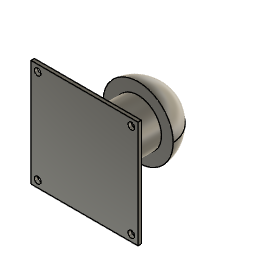
Suport+Topo+V2 (Autodesk Fusion 360 archive; units mm, degrees)
design "camera"
Autodesk Fusion 360 part; units mm, degrees
sketch "Sketch1" plane through (0, 0, 0) normal (0, 1, 0) x (1, 0, 0)
  line L0 (0, 0) -> (32, 0)
  line L1 (32, 0) -> (32, -32)
  line L2 (32, -32) -> (0, -32)
  line L3 (0, -32) -> (0, 0)
  circle A0 centre (1.6953, -30.2758) radius 1.5
  circle A1 centre (1.6953, -1.6758) radius 1.5
  circle A2 centre (30.3047, -30.2758) radius 1.5
  circle A3 centre (30.3047, -1.6758) radius 1.5
  line L4 (-1, -16) -> (38, -16)
  line L5 (0, -13) -> (9.5, -13)
  line L6 (32, -13) -> (22.5, -13)
  line L7 (9.5, 0.8661) -> (9.5, -33)
  line L8 (22.5, 0.9345) -> (22.5, -33)
  line L9 (16, 2.2342) -> (16, -35)
  line L10 (22.5, -9.5) -> (9.5, -9.5)
  line L11 (9.5, -9.5) -> (9.5, -22.5)
  line L12 (9.5, -22.5) -> (22.5, -22.5)
  line L13 (22.5, -22.5) -> (22.5, -9.5)
  line L14 (22.5, -9.5) -> (9.5, -22.5) construction
  line L15 (9.5, -9.5) -> (22.5, -22.5) construction
  circle A4 centre (16, -16) radius 6.5
  line L16 (0, 1) -> (10, 1)
  line L17 (32, 1) -> (20, 1)
  line L18 (10, 1) -> (10, -6)
  line L19 (20, 1) -> (20, -6)
  line L20 (10, -5.4961) -> (20, -5.4961)
  line L21 (20, -5.4961) -> (20, -0.4961)
  line L22 (20, -0.4961) -> (10, -0.4961)
  line L23 (10, -0.4961) -> (10, -5.4961)
  line L24 (24.5, -14) -> (22.5, -14)
  line L25 (22.5, -14) -> (22.5, -18)
  line L26 (22.5, -18) -> (24.5, -18)
  line L27 (24.5, -18) -> (24.5, -14)
  arc A5 (24.5, -18) -> (24.5, -14) centre (24.5, -16) ccw
  arc A6 (22.5, -15.9983) -> (22.5, -16.0017) centre (24.5, -16) ccw
  arc A7 (7.5, -14) -> (7.5, -18) centre (7.5, -16) ccw
  line L28 (7.5, -14) -> (9.5, -14)
  line L29 (9.5, -18) -> (7.5, -18)
  point P0 (16, -16)
  constraint horizontal L0
  constraint vertical L1
  constraint horizontal L2
  constraint vertical L3
  constraint coincident L0.start L3.end
  constraint coincident L3 L5.start
  constraint perpendicular L3 L5
  constraint coincident L1 L6.start
  constraint perpendicular L1 L6
  constraint perpendicular L2 L7
  constraint perpendicular L2 L8
  constraint perpendicular L2 L9
  constraint horizontal L10
  constraint perpendicular L10 L11
  constraint parallel L10 L12
  constraint parallel L11 L13
  constraint coincident L14 P0
  constraint coincident L15 P0
  constraint coincident L4 P0
  constraint coincident L9 P0
  constraint coincident P0 A4.centre
  constraint tangent L13 A4
  constraint perpendicular L3 L16
  constraint perpendicular L8 L17
  constraint perpendicular L0 L18
  constraint perpendicular L0 L19
  constraint horizontal L20
  constraint vertical L21
  constraint horizontal L22
  constraint vertical L23
  constraint coincident L18 L20.start
  constraint horizontal L24
  constraint vertical L25
  constraint horizontal L26
  constraint vertical L27
  constraint midpoint L27 A5.centre
  constraint coincident L8 A6.end
  constraint coincident L8 A6.start
  constraint concentric A5 A6
  constraint symmetric L9 L24.start A7.start
  constraint symmetric L9 L24.end L28.end
  constraint symmetric L9 L25.end L29.start
  constraint symmetric L9 L26.end A7.end
  constraint symmetric L9 A5 A7
extrude "Extrude1" add sketch "Sketch1" against normal blind 3 makes body 1
extrude "Extrude2" add sketch "Sketch1" along normal blind 12.5 contours L9 L18 L20 L22 L23 | L9 L19 L20 L21 L22 bodies 1
extrude "Extrude3" add sketch "Sketch1" against normal blind 6 contours L7 L10 L11 A4 | L4 L9 A4 | L8 L10 L13 A4 L25 | L4 L9 A4 | L4 L7 L11 A7 L28 | L4 L7 L11 A7 L29 | L4 L9 A4 | L4 L9 A4 | L4 L8 L13 L24 L25 L27 | L4 L8 L13 L25 L26 L27 | L8 L12 L13 A4 L25 | L7 L11 L12 A4 | L4 L27 A5 | L4 L27 A5 bodies 1
extrude "Extrude4" add sketch "Sketch1" against normal blind 18.4 contours L4 L9 A4 | L4 L9 A4 | L4 L9 A4 | L4 L9 A4 bodies 1
sketch "Sketch2" plane through (0, 0, 0) normal (0, 1, 0) x (1, 0, 0)
  circle A0 through (26.5, -16, -18.3) (10.75, -6.9067, -18.3) (10.75, -25.0933, -18.3)
extrude "Extrude5" add sketch "Sketch2" against normal blind 11 contours A0 in plane through (0, -18.3, 0) normal (0, 1, 0) bodies 1
sketch "Sketch3" plane through (0, 0, 0) normal (0, 1, 0) x (1, 0, 0)
  line L0 (0, 0) -> (-16, 0)
  line L1 (-16, 0) -> (-16, -16)
  line L2 (0, 0) -> (-32, 0)
  line L3 (-32, 0) -> (-32, -32)
  line L4 (-32, -32) -> (0, -32)
  line L5 (0, -32) -> (0, 0)
  line L6 (0, 0) -> (-32, -32) construction
  line L7 (-32, 0) -> (0, -32) construction
  line L8 (0, 0) -> (-2, 0)
  line L9 (-2, 0) -> (-2, -2)
  circle A0 centre (-2, -2) radius 1
  circle A1 centre (-30, -2) radius 1
  circle A2 centre (-30, -30) radius 1
  circle A3 centre (-2, -30) radius 1
  circle A4 centre (-16, -16) radius 7
  line L10 (-22.5, -9.5) -> (-9.5, -9.5)
  line L11 (-9.5, -9.5) -> (-9.5, -22.5)
  line L12 (-9.5, -22.5) -> (-22.5, -22.5)
  line L13 (-22.5, -22.5) -> (-22.5, -9.5)
  line L14 (-22.5, -9.5) -> (-9.5, -22.5) construction
  line L15 (-9.5, -9.5) -> (-22.5, -22.5) construction
  line L16 (-25.5, -14) -> (-18.5, -14)
  line L17 (-18.5, -14) -> (-18.5, -18)
  line L18 (-18.5, -18) -> (-25.5, -18)
  line L19 (-26.5, -17) -> (-26.5, -15)
  line L20 (-26.5, -14) -> (-18.5, -18) construction
  line L21 (-18.5, -14) -> (-26.5, -18) construction
  arc A5 (-26.5, -17) -> (-25.5, -18) centre (-25.5, -17) ccw
  arc A6 (-25.5, -14) -> (-26.5, -15) centre (-25.5, -15) ccw
  line L22 (-6.5, -18) -> (-13.5, -18)
  line L23 (-13.5, -18) -> (-13.5, -14)
  line L24 (-13.5, -14) -> (-6.5, -14)
  line L25 (-5.5, -15) -> (-5.5, -17)
  line L26 (-5.5, -18) -> (-13.5, -14) construction
  line L27 (-13.5, -18) -> (-5.5, -14) construction
  arc A7 (-6.5, -18) -> (-5.5, -17) centre (-6.5, -17) ccw
  arc A8 (-5.5, -15) -> (-6.5, -14) centre (-6.5, -15) ccw
  point P0 (-16, -16)
  point P1 (-16, -16)
  point P2 (-22.5, -16)
  point P3 (-9.5, -16)
  dimension "d25" = 16
  dimension "d26" = 16
  dimension "d27" = 2
  dimension "d28" = 2
  dimension "d30" = 360
  dimension "d31" = 14
  dimension "d32" = 13
  dimension "d33" = 13
  dimension "d34" = 8
  dimension "d35" = 4
  dimension "d40" = 1
  dimension "d41" = 1
  dimension "d53" = 8
  dimension "d54" = 4
  dimension "d55" = 1
  dimension "d56" = 1
  constraint coincident L0.start L2.start
  constraint horizontal L0
  constraint perpendicular L0 L1
  constraint horizontal L2
  constraint perpendicular L2 L3
  constraint parallel L2 L4
  constraint parallel L3 L5
  constraint coincident L6 P1
  constraint coincident L7 P1
  constraint coincident P1 P0
  constraint parallel L0 L8
  constraint coincident L6 L9.end
  constraint perpendicular L2 L9
  constraint coincident L9.end A0.centre
  constraint horizontal L10
  constraint perpendicular L10 L11
  constraint parallel L10 L12
  constraint parallel L11 L13
  constraint coincident L14 P1
  constraint coincident L15 P1
  constraint horizontal L16
  constraint perpendicular L16 L17
  constraint parallel L16 L18
  constraint parallel L17 L19
  constraint coincident L20 P2
  constraint coincident L21 P2
  constraint midpoint L13 P2
  constraint coincident L21.end L18
  constraint coincident L21.end L19
  constraint tangent L18 A5
  constraint tangent L19 A5
  constraint coincident L20.start L19
  constraint coincident L20.start L16
  constraint tangent L19 A6
  constraint tangent L16 A6
  constraint horizontal L22
  constraint perpendicular L22 L23
  constraint parallel L22 L24
  constraint parallel L23 L25
  constraint coincident L26 P3
  constraint coincident L27 P3
  constraint midpoint L11 P3
  constraint coincident L26.start L22
  constraint coincident L26.start L25
  constraint tangent L22 A7
  constraint tangent L25 A7
  constraint coincident L27.end L24
  constraint coincident L27.end L25
  constraint tangent L24 A8
  constraint tangent L25 A8
  measures "d25" distance of L0.start L0.end
  measures "d26" distance of L0.end P1
  measures "d27" distance of L0.start L8.end
  measures "d28" diameter of A0
  measures "d31" diameter of A4
  measures "d32" distance of L11.end L12.end
  measures "d33" distance of L10.end L11.end
  measures "d34" distance of L17.end L21.end
  measures "d35" distance of L16.end L17.end
  measures "d40" radius of A5
  measures "d41" radius of A6
  measures "d53" distance of L23.end L27.end
  measures "d54" distance of L22.end L23.end
  measures "d55" radius of A7
  measures "d56" radius of A8
extrude "Extrude6" add sketch "Sketch3" along normal blind 1 separate body contours L0 L2 L3 L4 L5 L8 | L1 A4 L10 | L1 A4 L10 | A4 L10 L11 L12 L13 L16 L17 L18 L22 L23 L24 | A4 L10 L11 | A4 L10 L13 | A4 L11 L24 | A4 L13 L16 | A4 L22 L24 L25 A7 A8 | A4 L11 L22 L24 | L11 L22 L23 L24 | A4 L13 L16 L18 | A4 L16 L18 L19 A5 A6 | L13 L16 L17 L18 | A4 L11 L22 | A4 L13 L18 | A4 L11 L12 | A4 L12 L13 | A4 L12 makes body 2
extrude "Extrude7" add sketch "Sketch3" against normal blind 3 contours L1 A4 L10 | L1 A4 L10 | A4 L10 L11 L12 L13 L16 L17 L18 L22 L23 L24 | A4 L10 L11 | A4 L10 L13 | A4 L11 L24 | A4 L13 L16 | A4 L22 L24 L25 A7 A8 | A4 L11 L22 L24 | L11 L22 L23 L24 | A4 L13 L16 L18 | A4 L16 L18 L19 A5 A6 | L13 L16 L17 L18 | A4 L11 L22 | A4 L13 L18 | A4 L11 L12 | A4 L12 L13 | A4 L12 bodies 2
extrude "Extrude8" add sketch "Sketch3" against normal blind 15 contours L1 A4 L10 | L1 A4 L10 | A4 L10 L11 L12 L13 L16 L17 L18 L22 L23 L24 | A4 L11 L24 | A4 L13 L16 | A4 L11 L22 L24 | L11 L22 L23 L24 | A4 L13 L16 L18 | L13 L16 L17 L18 | A4 L11 L22 | A4 L13 L18 | A4 L12 bodies 2
sketch "Sketch4" plane through (0, -15, 0) normal (0, -1, 0) x (1, 0, 0)
  circle A0 centre (-16, 16) radius 7
  circle A1 centre (-16, 16) radius 10.5
  dimension "d48" = 21
  constraint concentric A0 A1
  measures "d48" diameter of A1
extrude "Extrude9" add sketch "Sketch4" along normal blind 10 contours A0 | A1 bodies 2
fillet "Fillet1" radius 10 tangency weight 0.79029 1 edges at (-25.7894, -25, 12.203) on bodies 2
move_body "Move1" bodies 2 to x (-1, 0, 0) y (0, -1, 0) z (0, 0, 1) at (0, 1, 0)
hidden bodies 1
equation "d25 = ( 32 / 2 ) * 1 mm"
equation "d26 = ( 32 / 2 ) * 1 mm"

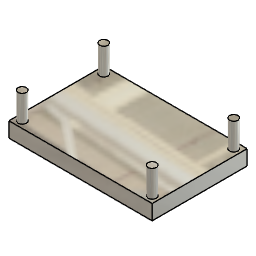
design "ecra Pi Pico"
Autodesk Fusion 360 part; units mm, degrees
sketch "Sketch1" plane through (0, 0, 0) normal (0, 1, 0) x (1, 0, 0)
  line L0 (43, -28.5) -> (-43, -28.5)
  line L1 (-43, -28.5) -> (-43, 28.5)
  line L2 (-43, 28.5) -> (43, 28.5)
  line L3 (43, 28.5) -> (43, -28.5)
  line L4 (43, -28.5) -> (-43, 28.5) construction
  line L5 (-43, -28.5) -> (43, 28.5) construction
  line L6 (43, -28.5) -> (39, -28.5)
  line L7 (39, -28.5) -> (39, -24.5)
  line L8 (39, -24.5) -> (43, -24.5)
  line L9 (43, -24.5) -> (43, -28.5)
  circle A0 centre (39, -24.5) radius 2.5
  line L10 (52.3114, 0) -> (-55.6196, 0)
  line L11 (0, 36.5366) -> (0, -32.8551)
  circle A1 centre (-39, -24.5) radius 2.5
  circle A2 centre (39, 24.5) radius 2.5
  circle A3 centre (-39, 24.5) radius 2.5
  dimension "d1" = 86
  dimension "d2" = 57
  dimension "d5" = 4
  dimension "d6" = 4
  dimension "d7" = 5
  constraint horizontal L0
  constraint perpendicular L0 L1
  constraint parallel L0 L2
  constraint parallel L1 L3
  constraint coincident L4 origin
  constraint coincident L5 origin
  constraint horizontal L6
  constraint vertical L7
  constraint horizontal L8
  constraint vertical L9
  constraint coincident L7.end L8.start
  constraint perpendicular L3 L10
  constraint vertical L11
  constraint symmetric A0 L11 A1
  constraint symmetric A0 L10 A2
  constraint symmetric L10 A1 A3
  measures "d1" distance of L1.end L2.end
  measures "d2" distance of L0.end L1.end
  measures "d5" distance of L0.start L6.end
  measures "d6" distance of L0.start L8.end
  measures "d7" diameter of A0
extrude "Extrude1" add sketch "Sketch1" along normal blind 9 contours L0 L3 L6 L7 L8 L9 A0 | L0 L3 L7 L8 A0 L10 L11 | L0 L1 L10 L11 | L7 L8 A0 | L7 L8 A0 | L2 L3 L10 L11 | L1 L2 L10 L11 | A1 | A2 | A3
extrude "Extrude2" add sketch "Sketch1" along normal blind 25 contours L7 L8 A0 | L7 L8 A0 | A1 | A2 | A3
